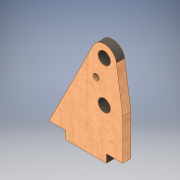
# Autodesk Inventor part: HolderSFC6
Saved by Autodesk Inventor 2019 (Build 230136000, 136)
## iProperties
Created: 2021-01-03
Part Number: HolderSFC6
Material: Дерево (вишня)
Document SubType Name: Modeling
Designer: Professional
Density: 0.63 g/cm^3
Appearance: Вишневое дерево — натуральный — со слабым глянцем
Author: Professional
Autodesk Inventor part; units mm, degrees
ref_plane "YZ Plane" through (0, 0, 0) normal (1, 0, 0) x (0, 1, 0)
ref_plane "XZ Plane" through (0, 0, 0) normal (0, 1, 0) x (-1, 0, 0)
ref_plane "XY Plane" through (0, 0, 0) normal (0, 0, 1) x (1, 0, 0)
sketch "Эскиз1" plane through (0, 0, 0) normal (0, 0, 1) x (1, 0, 0)
  line L0 (-20, 0) -> (-20, -4)
  line L1 (-20, -4) -> (0, -4)
  line L2 (0, -4) -> (0, 0)
  line L3 (0, 0) -> (8, 0)
  arc A0 (4.9364, 40.8714) -> (-6.3519, 42.7125) centre (-1, 40) ccw
  line L4 (-6.3519, 42.7125) -> (-28, 0)
  line L5 (-28, 0) -> (-20, 0)
  circle A1 centre (-1, 40) radius 3
  circle A2 centre (-1, 20) radius 3
  line L6 (8, 0) -> (8, 20)
  line L7 (8, 20) -> (4.9364, 40.8714)
  dimension "d0" = 6
  dimension "d1" = 40
  dimension "d2" = 20
  dimension "d3" = 4
  dimension "d4" = 20
  dimension "d5" = 6
  dimension "d14" = 1
  dimension "d15" = 20
  dimension "d16" = 36
  constraints: 16 end point, 3 centre point, 3 perpendicular, 2 coincident, 2 point on circle, 2 tangent, 2 vertical, 1 collinear, 1 equal radius, 1 horizontal, 1 horizontal alignment, 1 vertical alignment
  measures "d0" radius of A0
  measures "d1" distance from line of A0.centre L3
  measures "d2" distance of L0.end L1.end
  measures "d3" distance between parallel lines of L3 L1
  measures "d4" distance from line of L3 A2.centre
  measures "d5" diameter of A1
  measures "d14" distance from line of A2.centre L2
  measures "d15" distance of L3.end L6.end
  measures "d16" distance of L3.end L4.end
extrude "Выдавливание1" add sketch "Эскиз1" along normal blind 4
sketch "Эскиз2" plane through (0, 0, 4) normal (0, 0, 1) x (1, 0, 0)
  circle A0 centre (-5, 30) radius 1.5
  line L0 (0, 0) -> (8, 0) projected
  line L1 (8, 0) -> (8, 20) projected
  dimension "d9" = 3
  dimension "d10" = 30
  dimension "d17" = 13
  constraints: 1 centre point
  measures "d9" diameter of A0
  measures "d10" distance from line of L0 A0.centre
  measures "d17" distance from line of L1 A0.centre
extrude "Выдавливание2" cut sketch "Эскиз2" against normal through all
